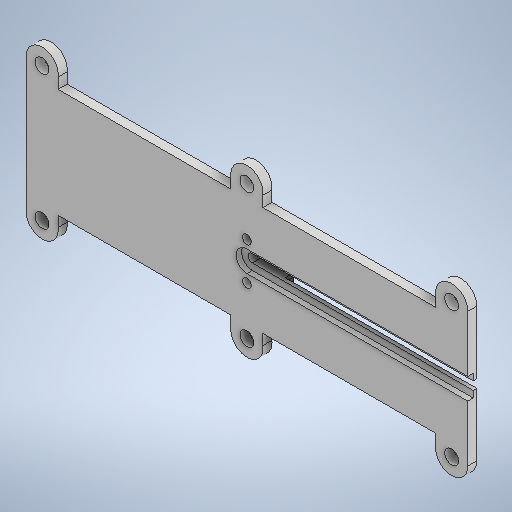
# Autodesk Inventor part: Gripper_BackPlate_Long
Saved by Autodesk Inventor 2025.1 (Build 291241000, 241)
## iProperties
Created: 2024-08-02
Part Number: Gripper_BackPlate_Long
Material: Generic
Document SubType Name: Modeling
Designer: leonh
Density: 1 g/cm^3
Appearance: Default
Author: leonh
Autodesk Inventor part; units mm, degrees
ref_plane "YZ Plane" through (0, 0, 0) normal (1, 0, 0) x (0, 1, 0)
ref_plane "XZ Plane" through (0, 0, 0) normal (0, 1, 0) x (-1, 0, 0)
ref_plane "XY Plane" through (0, 0, 0) normal (0, 0, 1) x (1, 0, 0)
sketch "Sketch1" plane through (0, 0, 0) normal (0, 0, 1) x (1, 0, 0)
  line L0 (-8.76, 11.0126) -> (-8.76, 0.5126)
  line L1 (-8.76, 0.5126) -> (-11.24, -14.9874)
  line L2 (-11.24, -14.9874) -> (8.76, -14.9874)
  line L3 (8.76, -14.9874) -> (8.76, -4.4874)
  line L4 (11.24, 11.0126) -> (-8.76, 11.0126)
  line L5 (0, 12.916) -> (0, -18.5653)
  line L6 (-8.76, 0.5126) -> (13.6474, 0.5126) construction
  line L7 (8.76, -4.4874) -> (-2.6872, -4.4874) construction
  line L8 (-5.8361, -1.9874) -> (18.6079, -1.9874) construction
  circle A0 centre (0, -7.7374) radius 1.325
  circle A1 centre (0, 3.7626) radius 1.325
  line L9 (22.7948, -1.9874) -> (0, -1.9874) construction
  line L10 (9.36, -0.7374) -> (0, -0.7374)
  line L11 (0, -3.2374) -> (8.96, -3.2374)
  arc A2 (0, -0.7374) -> (0, -3.2374) centre (0, -1.9874) ccw
  line L12 (8.76, -4.4874) -> (8.96, -3.2374)
  line L13 (9.36, -0.7374) -> (11.24, 11.0126)
  point P0 (0, 0)
  point P1 (-8.76, -4.4874)
  point P2 (11.3974, -1.9874)
  dimension "d0" = 2.48
  dimension "d1" = 15.5
  dimension "d2" = 15.5
  dimension "d3" = 2.48
  dimension "d4" = 10.5
  dimension "d5" = 10.5
  dimension "d6" = 20
  dimension "d7" = 20
  dimension "d8" = 2.65
  dimension "d9" = 7.25
  dimension "d12" = 2.5
  dimension "d26" = 11.75
  dimension "d27" = 14.25
  constraints: 30 end point, 4 point on line, 3 centre point, 2 horizontal, 2 perpendicular, 2 point on circle, 2 symmetric about line, 2 tangent, 2 vertical, 2 vertical alignment, 1 collinear, 1 midpoint, 1 parallel, 2 other
  measures "d0" horizontal distance of L1.end L0.end
  measures "d1" vertical distance of L1.end L0.end
  measures "d2" vertical distance of L4.start L3.end
  measures "d3" horizontal distance of L4.start L3.end
  measures "d4" distance of L0.start L0.end
  measures "d5" distance of L2.end L3.end
  measures "d6" distance of L4.start L0.start
  measures "d7" distance of L2.end L1.end
  measures "d8" diameter of A0
  measures "d9" distance from line of A0.centre L2
  measures "d12" diameter of A2
  measures "d26" vertical distance of L2.end L11.end
  measures "d27" vertical distance of L2.end L10.start
extrude "Extrusion1" add sketch "Sketch1" against normal blind 2.8 contours L4 L5 A1 A2 A0 L2 L1 L0 | L4 L13 L10 L5 A1 | L5 A0 L11 L12 L3 L2
sketch "Sketch2" plane through (0, 0, 0) normal (0, 0, 1) x (1, 0, 0)
  line L0 (-67.25, -18.5874) -> (-67.25, 14.6126)
  line L1 (0, 12.916) -> (0, -18.5653) construction
  line L2 (-5.8361, -1.9874) -> (18.6079, -1.9874) construction
  line L3 (-67.25, 14.6126) -> (-67.25, 18.4126)
  line L4 (-57.4847, 14.6126) -> (-57.4847, 17.8301)
  arc A0 (-57.4847, 17.8301) -> (-67.25, 18.4126) centre (-62.35, 18.4126) ccw
  line L5 (0, 12.916) -> (0, -18.5653)
  circle A1 centre (-62.35, 18.4126) radius 2.1
  arc A2 (0, -0.7374) -> (0, -3.2374) centre (0, -1.9874) ccw projected
  line L6 (-1.25, -1.9874) -> (17.7749, -1.9874) construction
  line L7 (0, -3.2374) -> (67.25, -3.2374)
  line L8 (67.25, -0.7374) -> (0, -0.7374)
  arc A3 (0, -0.7374) -> (0, -3.2374) centre (0, -1.9874) ccw
  line L9 (67.25, 14.6126) -> (67.25, -0.7374)
  line L10 (67.25, -3.2374) -> (67.25, -18.5874)
  line L11 (-4.9, -18.5874) -> (-24.8081, -18.5874)
  circle A4 centre (0, 3.7626) radius 1.325 projected
  circle A5 centre (0, -7.7374) radius 1.325 projected
  line L12 (67.25, 14.6126) -> (67.25, 18.4126)
  line L13 (57.4847, 14.6126) -> (57.4847, 17.8301)
  arc A6 (67.25, 18.4126) -> (57.4847, 17.8301) centre (62.35, 18.4126) ccw
  circle A7 centre (62.35, 18.4126) radius 2.1
  line L14 (-67.25, -18.5874) -> (-67.25, -22.3874)
  line L15 (-57.4847, -18.5874) -> (-57.4847, -21.8049)
  arc A8 (-67.25, -22.3874) -> (-57.4847, -21.8049) centre (-62.35, -22.3874) ccw
  circle A9 centre (-62.35, -22.3874) radius 2.1
  line L16 (57.4847, -18.5874) -> (57.4847, -21.8049)
  circle A10 centre (62.35, -22.3874) radius 2.1
  line L17 (67.25, -18.5874) -> (67.25, -22.3874)
  arc A11 (57.4847, -21.8049) -> (67.25, -22.3874) centre (62.35, -22.3874) ccw
  line L18 (-4.9, 14.6126) -> (-4.9, 18.4126)
  line L19 (4.8653, 14.6126) -> (4.8653, 17.8301)
  arc A12 (4.8653, 17.8301) -> (-4.9, 18.4126) centre (0, 18.4126) ccw
  circle A13 centre (0, 18.4126) radius 2.1
  line L20 (-57.4847, 14.6126) -> (-4.9, 14.6126)
  line L21 (4.8653, 14.6126) -> (57.4847, 14.6126)
  line L22 (-4.9, -18.5874) -> (-4.9, -22.3874)
  line L23 (4.8653, -18.5874) -> (4.8653, -21.8049)
  arc A14 (-4.9, -22.3874) -> (4.8653, -21.8049) centre (0, -22.3874) ccw
  circle A15 centre (0, -22.3874) radius 2.1
  line L24 (57.4847, -18.5874) -> (4.8653, -18.5874)
  line L25 (-4.9, -18.5874) -> (-57.4847, -18.5874)
  point P0 (0, 0)
  point P1 (8.2624, -1.9874)
  point P2 (67.25, 14.6126)
  point P3 (39.75, 14.6126)
  point P4 (67.25, -18.5874)
  dimension "d15" = 4.9
  dimension "d16" = 4.2
  dimension "d25" = 134.5
  dimension "d38" = 4.9
  dimension "d39" = 4.2
  constraints: 50 end point, 25 symmetric about line, 16 point on circle, 13 centre point, 6 coincident, 4 vertical, 3 parallel, 3 point on line, 2 horizontal, 2 tangent, 2 vertical alignment, 1 collinear, 1 midpoint, 9 other
  measures "d15" radius of A0
  measures "d16" diameter of A1
  measures "d25" distance between parallel lines of L0 L9
  measures "d38" radius of A12
  measures "d39" diameter of A13
extrude "Extrusion2" add sketch "Sketch2" along normal blind 2.75 contours L0 L3 A0 L4 L20 L18 A12 L19 L21 L13 A6 L12 L9 L8 A2 L7 L10 L17 A11 L16 L24 L23 A14 L22 L11 L25 L15 A8 L14
sketch "Sketch3" plane through (0, 0, 2.75) normal (0, 0, 1) x (1, 0, 0)
  arc A0 (0, -0.7374) -> (0, -3.2374) centre (0, -1.9874) ccw projected
  line L0 (0, -1.9874) -> (79.0333, -1.9874) construction
  line L1 (0, -5.2374) -> (79.0333, -5.2374)
  line L2 (79.0333, 1.2626) -> (0, 1.2626)
  arc A1 (0, 1.2626) -> (0, -5.2374) centre (0, -1.9874) ccw
  arc A2 (79.0333, -5.2374) -> (79.0333, 1.2626) centre (79.0333, -1.9874) ccw
  point P0 (0, 0)
  point P1 (39.5166, -1.9874)
  dimension "d20" = 3.25
  constraints: 8 end point, 4 point on circle, 4 tangent, 2 centre point, 1 horizontal, 1 midpoint, 1 parallel
  measures "d20" radius of A1
extrude "Extrusion3" cut sketch "Sketch3" against normal blind 1.65
sketch "Sketch4" plane through (0, 0, 0) normal (0, 0, -1) x (-1, 0, 0)
  line L0 (-62.15, 8.0126) -> (-60.65, 8.0126)
  line L1 (-60.65, 8.0126) -> (-60.65, -0.7874)
  line L2 (-60.65, -0.7874) -> (-62.15, -0.7874)
  line L3 (-62.15, -0.7874) -> (-62.15, 8.0126)
  line L4 (-67.25, -0.7374) -> (-67.25, 18.4126) projected
  line L5 (-57.4847, 14.6126) -> (57.4847, 14.6126) projected
  line L6 (60.65, -3.1874) -> (62.15, -3.1874)
  line L7 (62.15, -3.1874) -> (62.15, -11.9874)
  line L8 (62.15, -11.9874) -> (60.65, -11.9874)
  line L9 (60.65, -11.9874) -> (60.65, -3.1874)
  line L10 (67.25, 18.4126) -> (67.25, -22.3874) projected
  line L11 (57.4847, -18.5874) -> (-57.4847, -18.5874) projected
  point P0 (0, 0)
  point P1 (-67.25, 8.8376)
  dimension "d28" = 5.1
  dimension "d29" = 6.6
  dimension "d30" = 8.8
  dimension "d31" = 1.5
  dimension "d32" = 5.1
  dimension "d34" = 8.8
  dimension "d35" = 1.5
  constraints: 16 end point, 4 parallel, 2 horizontal, 2 perpendicular, 1 midpoint
  measures "d28" distance from line of point (-67.25, 8.838) L3
  measures "d29" distance between parallel lines of L5 L0
  measures "d30" distance of L2.end L0.start
  measures "d31" distance between parallel lines of L1 L3
  measures "d32" distance between parallel lines of L10 L7
  measures "d34" distance between parallel lines of L8 L6
  measures "d35" distance between parallel lines of L7 L9
extrude "Extrusion4" add sketch "Sketch4" along normal blind 2.3
body "Solid1"
